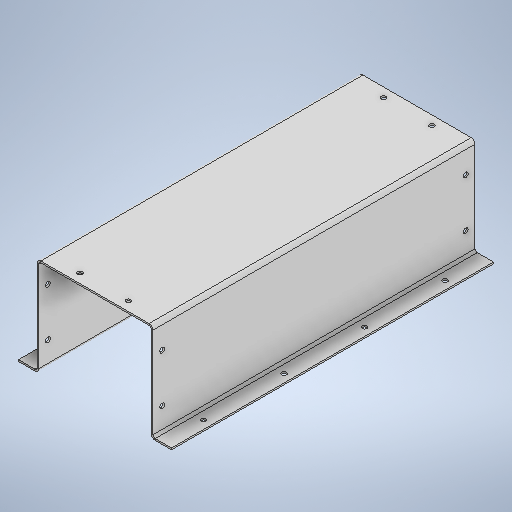
# Autodesk Inventor part: Кожух
Saved by Autodesk Inventor 2025 (Build 290162010, 162A)
## iProperties
Created: 2024-07-07
Part Number: Кожух
Material: Stainless Steel
Document SubType Name: Sheet Metal
Designer: pokla
Density: 8 g/cm^3
Sheet Metal Rule: AISI304 2mm Die16
Appearance: Default
Flat Pattern Width: 40 cm
Flat Pattern Length: 42.2808 cm
Flat Pattern Area: 1691.23 cm^2
Sheet Metal Width: 400,000 mm
Sheet Metal Length: 422,808 mm
Sheet Metal Area: 169123,185 mm^2
Author: pokla
Autodesk Inventor part; units mm, degrees
ref_plane "YZ Plane" through (0, 0, 0) normal (1, 0, 0) x (0, 1, 0)
ref_plane "XZ Plane" through (0, 0, 0) normal (0, 1, 0) x (-1, 0, 0)
ref_plane "XY Plane" through (0, 0, 0) normal (0, 0, 1) x (1, 0, 0)
sketch "Sketch1" plane through (0, 0, 0) normal (0, 0, 1) x (1, 0, 0)
  line L0 (-70, 200) -> (70, 200)
  line L1 (70, 200) -> (70, -200)
  line L2 (70, -200) -> (-70, -200)
  line L3 (-70, -200) -> (-70, 200)
  line L4 (-70, 200) -> (70, -200) construction
  point P0 (0, 0)
  point P1 (0, 0)
  dimension "d0" = 140
  dimension "d1" = 400
  measures "d0" distance of L0.start L0.end
  measures "d1" distance of L2.end L0.start
extrude "Plate1" add sketch "Sketch1" along normal blind 2
sketch "Sketch2" plane through (72, -200, 2) normal (-1, 0, 0) x (0, -1, 0)
  line L0 (-400, 0) -> (0, 0)
  line L1 (0, 0) -> (0, -120)
  line L2 (0, -120) -> (-400, -120)
  line L3 (-400, -120) -> (-400, 0)
  constraints: 8 end point
edge flange "Flange1" height 120 angle 90 thickness 2 bend radius 2.75 thickness toward (-1, 0, 0) relief round relief width 2 relief depth 1 edges at (70, 0, 0) wall of the first edge with corners at (72, 200, 2) (72, -200, 2) (72, -200, -118) (72, 200, -118)
bend "Bend1"
corner "Corner1"
sketch "Sketch3" plane through (-72, 200, 2) normal (1, 0, 0) x (0, 1, 0)
  line L0 (-400, 0) -> (0, 0)
  line L1 (0, 0) -> (0, -120)
  line L2 (0, -120) -> (-400, -120)
  line L3 (-400, -120) -> (-400, 0)
  constraints: 8 end point
edge flange "Flange2" height 120 angle 90 thickness 2 bend radius 2.75 thickness toward (1, 0, 0) relief round relief width 2 relief depth 1 edges at (-70, 0, 0) wall of the first edge with corners at (-72, -200, 2) (-72, 200, 2) (-72, 200, -118) (-72, -200, -118)
bend "Bend2"
corner "Corner2"
sketch "Sketch4" plane through (70, 200, -120) normal (0, 0, 1) x (1, 0, 0)
  line L0 (0, -400) -> (0, 0)
  line L1 (0, 0) -> (25, 0)
  line L2 (25, 0) -> (25, -400)
  line L3 (25, -400) -> (0, -400)
  constraints: 8 end point
edge flange "Flange3" height 25 angle 90 thickness 2 bend radius 2.75 thickness toward (0, 0, 1) relief round relief width 2 relief depth 1 edges at (72, 0, -118) wall of the first edge with corners at (70, -200, -120) (70, 200, -120) (95, 200, -120) (95, -200, -120)
bend "Bend3"
corner "Corner3"
sketch "Sketch5" plane through (-70, -200, -120) normal (0, 0, 1) x (1, 0, 0)
  line L0 (0, 400) -> (0, 0)
  line L1 (0, 0) -> (-25, 0)
  line L2 (-25, 0) -> (-25, 400)
  line L3 (-25, 400) -> (0, 400)
  constraints: 8 end point
edge flange "Flange4" height 25 angle 90 thickness 2 bend radius 2.75 thickness toward (0, 0, 1) relief round relief width 2 relief depth 1 edges at (-72, 0, -118) wall of the first edge with corners at (-70, 200, -120) (-70, -200, -120) (-95, -200, -120) (-95, 200, -120)
bend "Bend4"
corner "Corner4"
sketch "Sketch6" plane through (95, -200, -118) normal (0, 0, 1) x (1, 0, 0)
  circle A0 centre (-10.125, 350) radius 3
  line L0 (-20.25, 400) -> (0, 400) projected
  point P0 (-95, 200)
  point P1 (-10.125, 400)
  dimension "d43" = 6
  dimension "d44" = 50
  constraints: 1 centre point, 1 midpoint, 1 vertical alignment
  measures "d43" diameter of A0
  measures "d44" distance of A0.centre point (-10.125, 400)
extrude "Extrusion1" cut sketch "Sketch6" against normal through all
pattern_linear "Rectangular Pattern2" count 4 spacing 100 along (0, -1, 0) count 2 spacing 169.75 along (-1, 0, 0) of "Extrusion1"
sketch "Sketch8" plane through (72, -200, -2.75) normal (1, 0, 0) x (0, 0, -1)
  line L0 (0, 400) -> (112.5, 400) projected
  line L1 (117.25, 0) -> (117.25, 400) projected
  circle A0 centre (87.25, 388.5) radius 3
  circle A1 centre (27.25, 388.5) radius 3
  point P0 (-2.75, 200)
  dimension "d68" = 6
  dimension "d69" = 60
  dimension "d78" = 30
  dimension "d79" = 11.5
  constraints: 2 centre point, 1 equal radius, 1 horizontal alignment
  measures "d68" diameter of A0
  measures "d69" distance of A0.centre A1.centre
  measures "d78" distance from line of L1 A0.centre
  measures "d79" distance from line of L0 A0.centre
extrude "Extrusion3" cut sketch "Sketch8" against normal through all
sketch "Sketch9" plane through (0, 0, 2) normal (0, 0, 1) x (1, 0, 0)
  circle A0 centre (-29.95, 188.5) radius 3
  line L0 (-67.25, 200) -> (67.25, 200) projected
  line L1 (-67.25, 200) -> (-67.25, -200) projected
  circle A1 centre (30.05, 188.5) radius 3
  point P0 (0, 0)
  point P1 (67.25, 200)
  dimension "d72" = 6
  dimension "d73" = 11.5
  dimension "d74" = 37.3
  dimension "d80" = 60
  constraints: 2 centre point, 1 equal radius, 1 horizontal alignment, 1 other
  measures "d72" diameter of A0
  measures "d74" distance from line of L1 A0.centre
  measures "d80" distance of A1.centre A0.centre
extrude "Extrusion4" cut sketch "Sketch9" against normal through all
mirror "Mirror2" about plane through (0, 0, 0) normal (0, 1, 0) of "Extrusion3", "Extrusion4"
equation "\"d0\" = Ширина_крепления_корпуса"
equation "\"d1\" = Длина_базовой_пластины"
equation "\"d69\" = 0.5 * Длина_крепления_корпуса"
equation "\"d2\" = Thickness"
equation "\"d3\" = BendReliefWidth"
equation "\"d4\" = BendReliefDepth"
equation "\"d5\" = MinimumRemnant"
equation "\"d6\" = TransitionRadius"
equation "\"d7\" = Длина_крепления_корпуса"
equation "\"d9\" = BendRadius"
equation "\"d10\" = CornerReliefSize"
equation "\"d11\" = GapSize"
equation "\"d12\" = JacobiRadiusSize"
equation "\"d13\" = BendReliefWidth"
equation "\"d14\" = BendReliefDepth"
equation "\"d15\" = MinimumRemnant"
equation "\"d16\" = TransitionRadius"
equation "\"d17\" = Длина_крепления_корпуса"
equation "\"d19\" = BendRadius"
equation "\"d20\" = CornerReliefSize"
equation "\"d21\" = GapSize"
equation "\"d22\" = JacobiRadiusSize"
equation "\"d23\" = BendReliefWidth"
equation "\"d24\" = BendReliefDepth"
equation "\"d25\" = MinimumRemnant"
equation "\"d26\" = TransitionRadius"
equation "\"d29\" = BendRadius"
equation "\"d30\" = CornerReliefSize"
equation "\"d31\" = GapSize"
equation "\"d32\" = JacobiRadiusSize"
equation "\"d33\" = BendReliefWidth"
equation "\"d34\" = BendReliefDepth"
equation "\"d35\" = MinimumRemnant"
equation "\"d36\" = TransitionRadius"
equation "\"d39\" = BendRadius"
equation "\"d40\" = CornerReliefSize"
equation "\"d41\" = GapSize"
equation "\"d42\" = JacobiRadiusSize"
equation "\"BendReliefWidth\" = Thickness"
equation "\"BendReliefDepth\" = 0.5 * Thickness"
equation "\"CornerReliefSize\" = 4 * Thickness"
equation "\"MinimumRemnant\" = 2 * Thickness"
equation "\"TransitionRadius\" = BendRadius"
equation "\"JacobiRadiusSize\" = BendRadius"
equation "\"GapSize\" = Thickness"
equation "\"Ширина_крепления_корпуса\" = 140"
equation "\"Длина_базовой_пластины\" = 400"
equation "\"Длина_крепления_корпуса\" = 120"
equation "\"Thickness\" = 2"
equation "\"BendRadius\" = 2.75"
body "Solid1"
